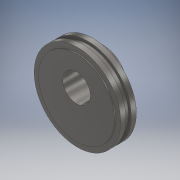
# Autodesk Inventor part: eccentric
Saved by Autodesk Inventor 2017 (Build 210142000, 142)
## iProperties
Created: 2018-11-11
Part Number: eccentric
Material: Steel, Alloy
Document SubType Name: Modeling
Designer: Arman Grewal
Density: 7.73 g/cm^3
Appearance: Semi-Polished
Author: Arman Grewal
Autodesk Inventor part; units mm, degrees
ref_plane "XZ Plane" through (0, 0, 0) normal (0, 1, 0) x (-1, 0, 0)
ref_plane "XY Plane" through (0, 0, 0) normal (0, 0, 1) x (1, 0, 0)
sketch "Sketch1" plane through (0, 0, 0) normal (0, 1, 0) x (-1, 0, 0)
  circle A0 centre (0, 0) radius 11
  dimension "d0" = 22
  constraints: 1 centre point, 1 coincident
  measures "d0" diameter of A0
extrude "Extrusion1" add sketch "Sketch1" along normal blind 0.25
sketch "Sketch2" plane through (0, 0.25, 0) normal (0, 1, 0) x (1, 0, 0)
  circle A0 centre (0, 0) radius 12.5
  dimension "d3" = 25
  constraints: 1 centre point, 1 coincident
  measures "d3" diameter of A0
extrude "Extrusion2" add sketch "Sketch2" along normal blind 1.5
sketch "Sketch3" plane through (0, 1.75, 0) normal (0, 1, 0) x (1, 0, 0)
  circle A0 centre (0, 0) radius 11.75
  dimension "d6" = 23.5
  constraints: 1 centre point, 1 coincident
  measures "d6" diameter of A0
extrude "Extrusion3" add sketch "Sketch3" along normal blind 1.5
sketch "Sketch4" plane through (0, 3.25, 0) normal (0, 1, 0) x (1, 0, 0)
  circle A0 centre (0, 0) radius 12.5
  dimension "d9" = 25
  constraints: 1 centre point, 1 coincident
  measures "d9" diameter of A0
extrude "Extrusion4" add sketch "Sketch4" along normal blind 1.5
sketch "Sketch5" plane through (0, 4.75, 0) normal (0, 1, 0) x (1, 0, 0)
  line L0 (0, 0) -> (0, -2.5) construction
  circle A0 centre (0, -2.5) radius 6.75 construction
  circle A1 centre (0, -2.5) radius 6.75
  circle A2 centre (0, -2.5) radius 4
  dimension "d12" = 2.5
  dimension "d13" = 13.5
  dimension "d14" = 8
  dimension "d15" = 13.5
  constraints: 3 centre point, 3 coincident, 2 end point, 1 vertical
  measures "d12" distance of L0.start L0.end
  measures "d13" diameter of A0
  measures "d14" diameter of A2
  measures "d15" diameter of A1
extrude "Extrusion5" add sketch "Sketch5" along normal blind 3
sketch "Sketch6" plane through (0, 4.75, 2.5) normal (0, 1, 0) x (1, 0, 0)
  circle A0 centre (0, 0) radius 4
  line L0 (0, 0) -> (-12.2474, 0) construction
  circle A1 centre (0, 2.5) radius 12.5 construction
  dimension "d18" = 8
  dimension "d19" = 2.5
  dimension "d20" = 12.2475
  constraints: 2 end point, 1 centre point, 1 horizontal, 2 other
  measures "d18" diameter of A0
  measures "d19" distance of point (0, 2.5) L0.start
  measures "d20" distance of L0.end L0.start
extrude "Extrusion6" cut sketch "Sketch6" against normal blind 999
ref_plane "Work Plane2" through (-10.25, 0, 0) normal (1, 0, 0) x (0, 1, 0)
sketch "Sketch8" plane through (-10.25, 0, 0) normal (1, 0, 0) x (0, 1, 0)
  line L0 (7.75, -4.25) -> (7.75, 9.25) construction
  line L1 (7.75, 0) -> (4.75, 0) construction
  line L2 (4.75, 9.25) -> (4.75, -4.25) construction
  line L3 (6.25, 0) -> (6.25, 7.0333) construction
  line L4 (7.75, 2.5) -> (4.75, 2.5) construction
  circle A0 centre (6.25, 2.5) radius 1.5
  point P0 (0, 0)
  dimension "d25" = 3
  dimension "d26" = 3
  constraints: 6 end point, 4 midpoint, 2 point on line, 1 centre point, 1 vertical
  measures "d25" distance of L1.start L1.end
  measures "d26" diameter of A0
extrude "Extrusion7" cut sketch "Sketch8" along normal blind 9
thread "Thread1" size "M2.5x0.45" class "6H" standard "ANSI Metric M Profile" length 6
body "Solid1"
